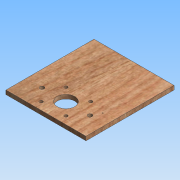
# Autodesk Inventor part: holder_plate
Saved by Autodesk Inventor 2015 (Build 190159000, 159)
## iProperties
Created: 2013-12-24
Part Number: holder_plate
Material: Wood (Birch)
Document SubType Name: Modeling
Designer: aoki
Density: 1 g/cm^3
Appearance: Birch - Natural Polished
Author: aoki
Autodesk Inventor part; units mm, degrees
ref_plane "YZ Plane" through (0, 0, 0) normal (1, 0, 0) x (0, 1, 0)
ref_plane "XZ Plane" through (0, 0, 0) normal (0, 1, 0) x (-1, 0, 0)
ref_plane "XY Plane" through (0, 0, 0) normal (0, 0, 1) x (1, 0, 0)
sketch "Block1" plane through (0, 0, 0) normal (0, 0, 1) x (1, 0, 0)
  line L0 (-30.1, 34.1) -> (-9.9, 34.1)
  line L1 (-9.9, 34.1) -> (-9.9, 25.1)
  line L2 (-9.9, 25.1) -> (9.9, 25.1)
  line L3 (9.9, 25.1) -> (9.9, 34.1)
  line L4 (9.9, 34.1) -> (30.1, 34.1)
  line L5 (30.1, 34.1) -> (30.1, 25.1)
  line L6 (30.1, 25.1) -> (50.1, 25.1)
  line L7 (50.1, 25.1) -> (50.1, 16.5667)
  line L8 (50.1, 16.5667) -> (41.1, 16.5667)
  line L9 (41.1, 16.5667) -> (41.1, 6.7667)
  line L10 (41.1, 6.7667) -> (50.1, 6.7667)
  line L11 (50.1, 6.7667) -> (50.1, -6.7667)
  line L12 (50.1, -6.7667) -> (41.1, -6.7667)
  line L13 (41.1, -6.7667) -> (41.1, -16.5667)
  line L14 (41.1, -16.5667) -> (50.1, -16.5667)
  line L15 (50.1, -16.5667) -> (50.1, -25.1)
  line L16 (50.1, -25.1) -> (30.1, -25.1)
  line L17 (30.1, -25.1) -> (30.1, -34.1)
  line L18 (30.1, -34.1) -> (9.9, -34.1)
  line L19 (9.9, -34.1) -> (9.9, -25.1)
  line L20 (9.9, -25.1) -> (-9.9, -25.1)
  line L21 (-9.9, -25.1) -> (-9.9, -34.1)
  line L22 (-9.9, -34.1) -> (-30.1, -34.1)
  line L23 (-30.1, -34.1) -> (-30.1, -25.1)
  line L24 (-30.1, -25.1) -> (-50.1, -25.1)
  line L25 (-50.1, -25.1) -> (-50.1, -16.5667)
  line L26 (-50.1, -16.5667) -> (-41.1, -16.5667)
  line L27 (-41.1, -16.5667) -> (-41.1, -6.7667)
  line L28 (-41.1, -6.7667) -> (-50.1, -6.7667)
  line L29 (-50.1, -6.7667) -> (-50.1, 6.7667)
  line L30 (-50.1, 6.7667) -> (-41.1, 6.7667)
  line L31 (-41.1, 6.7667) -> (-41.1, 16.5667)
  line L32 (-41.1, 16.5667) -> (-50.1, 16.5667)
  line L33 (-50.1, 16.5667) -> (-50.1, 25.1)
  line L34 (-50.1, 25.1) -> (-30.1, 25.1)
  line L35 (-30.1, 25.1) -> (-30.1, 34.1)
  circle A0 centre (-30, 0) radius 4.6
  circle A1 centre (-15.5, 15.5) radius 2.1
  circle A2 centre (-15.5, -15.5) radius 2.1
  circle A3 centre (0, 0) radius 11.1
  circle A4 centre (15.5, 15.5) radius 2.1
  circle A5 centre (30, 0) radius 4.6
  circle A6 centre (15.5, -15.5) radius 2.1
  point P0 (0, 0)
sketch "Block2" plane through (0, 0, 0) normal (0, 0, 1) x (1, 0, 0)
  line L0 (9.8, 34.2) -> (30.2, 34.2)
  line L1 (30.2, 34.2) -> (30.2, 25.2)
  line L2 (30.2, 25.2) -> (50.2, 25.2)
  line L3 (50.2, 25.2) -> (50.2, 16.4667)
  line L4 (50.2, 16.4667) -> (41.2, 16.4667)
  line L5 (41.2, 16.4667) -> (41.2, 6.8667)
  line L6 (41.2, 6.8667) -> (50.2, 6.8667)
  line L7 (50.2, 6.8667) -> (50.2, -6.8667)
  line L8 (50.2, -6.8667) -> (41.2, -6.8667)
  line L9 (41.2, -6.8667) -> (41.2, -16.4667)
  line L10 (41.2, -16.4667) -> (50.2, -16.4667)
  line L11 (50.2, -16.4667) -> (50.2, -25.2)
  line L12 (50.2, -25.2) -> (30.2, -25.2)
  line L13 (30.2, -25.2) -> (30.2, -34.2)
  line L14 (30.2, -34.2) -> (9.8, -34.2)
  line L15 (9.8, -34.2) -> (9.8, -25.2)
  line L16 (9.8, -25.2) -> (-9.8, -25.2)
  line L17 (-9.8, -25.2) -> (-9.8, -34.2)
  line L18 (-9.8, -34.2) -> (-30.2, -34.2)
  line L19 (-30.2, -34.2) -> (-30.2, -25.2)
  line L20 (-30.2, -25.2) -> (-50.2, -25.2)
  line L21 (-50.2, -25.2) -> (-50.2, -16.4667)
  line L22 (-50.2, -16.4667) -> (-41.2, -16.4667)
  line L23 (-41.2, -16.4667) -> (-41.2, -6.8667)
  line L24 (-41.2, -6.8667) -> (-50.2, -6.8667)
  line L25 (-50.2, -6.8667) -> (-50.2, 6.8667)
  line L26 (-50.2, 6.8667) -> (-41.2, 6.8667)
  line L27 (-41.2, 6.8667) -> (-41.2, 16.4667)
  line L28 (-41.2, 16.4667) -> (-50.2, 16.4667)
  line L29 (-50.2, 16.4667) -> (-50.2, 25.2)
  line L30 (-50.2, 25.2) -> (-30.2, 25.2)
  line L31 (-30.2, 25.2) -> (-30.2, 34.2)
  line L32 (-30.2, 34.2) -> (-9.8, 34.2)
  line L33 (-9.8, 34.2) -> (-9.8, 25.2)
  line L34 (-9.8, 25.2) -> (9.8, 25.2)
  line L35 (9.8, 25.2) -> (9.8, 34.2)
  circle A0 centre (-15.5, 15.5) radius 2.2
  circle A1 centre (15.5, 15.5) radius 2.2
  circle A2 centre (30, 0) radius 4.7
  circle A3 centre (15.5, -15.5) radius 2.2
  circle A4 centre (-15.5, -15.5) radius 2.2
  circle A5 centre (-30, 0) radius 4.7
  circle A6 centre (0, 0) radius 11.2
  point P0 (0, 0)
sketch "Block3" plane through (0, 0, 0) normal (0, 0, 1) x (1, 0, 0)
  line L0 (9.9, 34.1) -> (30.1, 34.1)
  line L1 (30.1, 34.1) -> (30.1, 25.1)
  line L2 (30.1, 25.1) -> (50.1, 25.1)
  line L3 (50.1, 25.1) -> (50.1, 16.5667)
  line L4 (50.1, 16.5667) -> (41.1, 16.5667)
  line L5 (41.1, 16.5667) -> (41.1, 6.7667)
  line L6 (41.1, 6.7667) -> (50.1, 6.7667)
  line L7 (50.1, 6.7667) -> (50.1, -6.7667)
  line L8 (50.1, -6.7667) -> (41.1, -6.7667)
  line L9 (41.1, -6.7667) -> (41.1, -16.5667)
  line L10 (41.1, -16.5667) -> (50.1, -16.5667)
  line L11 (50.1, -16.5667) -> (50.1, -25.1)
  line L12 (50.1, -25.1) -> (30.1, -25.1)
  line L13 (30.1, -25.1) -> (30.1, -34.1)
  line L14 (30.1, -34.1) -> (9.9, -34.1)
  line L15 (9.9, -34.1) -> (9.9, -25.1)
  line L16 (9.9, -25.1) -> (-9.9, -25.1)
  line L17 (-9.9, -25.1) -> (-9.9, -34.1)
  line L18 (-9.9, -34.1) -> (-30.1, -34.1)
  line L19 (-30.1, -34.1) -> (-30.1, -25.1)
  line L20 (-30.1, -25.1) -> (-50.1, -25.1)
  line L21 (-50.1, -25.1) -> (-50.1, -16.5667)
  line L22 (-50.1, -16.5667) -> (-41.1, -16.5667)
  line L23 (-41.1, -16.5667) -> (-41.1, -6.7667)
  line L24 (-41.1, -6.7667) -> (-50.1, -6.7667)
  line L25 (-50.1, -6.7667) -> (-50.1, 6.7667)
  line L26 (-50.1, 6.7667) -> (-41.1, 6.7667)
  line L27 (-41.1, 6.7667) -> (-41.1, 16.5667)
  line L28 (-41.1, 16.5667) -> (-50.1, 16.5667)
  line L29 (-50.1, 16.5667) -> (-50.1, 25.1)
  line L30 (-50.1, 25.1) -> (-30.1, 25.1)
  line L31 (-30.1, 25.1) -> (-30.1, 34.1)
  line L32 (-30.1, 34.1) -> (-9.9, 34.1)
  line L33 (-9.9, 34.1) -> (-9.9, 25.1)
  line L34 (-9.9, 25.1) -> (9.9, 25.1)
  line L35 (9.9, 25.1) -> (9.9, 34.1)
  circle A0 centre (-15.5, 15.5) radius 2.1
  circle A1 centre (15.5, 15.5) radius 2.1
  circle A2 centre (30, 0) radius 4.6
  circle A3 centre (15.5, -15.5) radius 2.1
  circle A4 centre (-15.5, -15.5) radius 2.1
  circle A5 centre (-30, 0) radius 4.6
  circle A6 centre (0, 0) radius 11.1
  point P0 (0, 0)
sketch "Block4" plane through (0, 0, 0) normal (0, 0, 1) x (1, 0, 0)
  line L0 (-30.08, 30.58) -> (-9.92, 30.58)
  line L1 (-9.92, 30.58) -> (-9.92, 25.08)
  line L2 (-9.92, 25.08) -> (9.92, 25.08)
  line L3 (9.92, 25.08) -> (9.92, 30.58)
  line L4 (9.92, 30.58) -> (30.08, 30.58)
  line L5 (30.08, 30.58) -> (30.08, 25.08)
  line L6 (30.08, 25.08) -> (50.08, 25.08)
  line L7 (50.08, 25.08) -> (50.08, 16.5867)
  line L8 (50.08, 16.5867) -> (44.58, 16.5867)
  line L9 (44.58, 16.5867) -> (44.58, 6.7467)
  line L10 (44.58, 6.7467) -> (50.08, 6.7467)
  line L11 (50.08, 6.7467) -> (50.08, -6.7467)
  line L12 (50.08, -6.7467) -> (44.58, -6.7467)
  line L13 (44.58, -6.7467) -> (44.58, -16.5867)
  line L14 (44.58, -16.5867) -> (50.08, -16.5867)
  line L15 (50.08, -16.5867) -> (50.08, -25.08)
  line L16 (50.08, -25.08) -> (30.08, -25.08)
  line L17 (30.08, -25.08) -> (30.08, -30.58)
  line L18 (30.08, -30.58) -> (9.92, -30.58)
  line L19 (9.92, -30.58) -> (9.92, -25.08)
  line L20 (9.92, -25.08) -> (-9.92, -25.08)
  line L21 (-9.92, -25.08) -> (-9.92, -30.58)
  line L22 (-9.92, -30.58) -> (-30.08, -30.58)
  line L23 (-30.08, -30.58) -> (-30.08, -25.08)
  line L24 (-30.08, -25.08) -> (-50.08, -25.08)
  line L25 (-50.08, -25.08) -> (-50.08, -16.5867)
  line L26 (-50.08, -16.5867) -> (-44.58, -16.5867)
  line L27 (-44.58, -16.5867) -> (-44.58, -6.7467)
  line L28 (-44.58, -6.7467) -> (-50.08, -6.7467)
  line L29 (-50.08, -6.7467) -> (-50.08, 6.7467)
  line L30 (-50.08, 6.7467) -> (-44.58, 6.7467)
  line L31 (-44.58, 6.7467) -> (-44.58, 16.5867)
  line L32 (-44.58, 16.5867) -> (-50.08, 16.5867)
  line L33 (-50.08, 16.5867) -> (-50.08, 25.08)
  line L34 (-50.08, 25.08) -> (-30.08, 25.08)
  line L35 (-30.08, 25.08) -> (-30.08, 30.58)
  circle A0 centre (-30, 0) radius 4.88
  circle A1 centre (30, 0) radius 4.88
  circle A2 centre (15.5, 15.5) radius 2.08
  circle A3 centre (0, 0) radius 11.08
  circle A4 centre (-15.5, 15.5) radius 2.08
  circle A5 centre (-15.5, -15.5) radius 2.08
  circle A6 centre (15.5, -15.5) radius 2.08
  point P0 (0, 0)
sketch "Sketch10" plane through (0, 0, 0) normal (0, 0, 1) x (1, 0, 0)
  line L0 (50, -25) -> (-50, -25)
  line L1 (-50, -25) -> (-50, 25)
  line L2 (-50, 25) -> (50, 25)
  line L3 (50, 25) -> (50, -25)
  line L4 (50, -25) -> (-50, 25) construction
  line L5 (-50, -25) -> (50, 25) construction
  point P0 (0, 0)
  dimension "d21" = 100
  dimension "d22" = 50
  constraints: 12 end point, 2 midpoint, 2 parallel, 1 horizontal, 1 perpendicular
  measures "d21" distance of L1.end L2.end
  measures "d22" distance of L0.end L1.end
extrude "Extrusion2" add sketch "Sketch10" against normal blind 5
sketch "Sketch13" plane through (0, 0, 0) normal (0, 0, 1) x (1, 0, 0)
  line L0 (0, -47.8822) -> (0, 48.5933) projected
  line L1 (-201.8331, 0) -> (92.0889, 0) projected
  point P0 (-15.5, 15.5)
  point P1 (15.5, 15.5)
  point P2 (-15.5, -15.5)
  point P3 (15.5, -15.5)
  dimension "d43" = 31
  dimension "d44" = 31
  constraints: 3 symmetric about line
  measures "d43" distance of point (15.5, 15.5) point (-15.5, 15.5)
  measures "d44" distance of point (-15.5, -15.5) point (-15.5, 15.5)
hole "Hole4" at (-15.5, 15.5, 0) at (15.5, 15.5, 0) at (-15.5, -15.5, 0) at (15.5, -15.5, 0) direction (0, 0, -1) diameter 4 end through all
sketch "Sketch16" plane through (0, 0, -5) normal (0, 0, -1) x (-1, 0, 0)
  line L0 (0, -47.8822) -> (0, 48.5933) projected
  point P0 (0, 0)
  point P1 (-30, 0)
  point P2 (30, 0)
  dimension "d52" = 60
  constraints: 1 symmetric about line
  measures "d52" distance of point (30, 0) point (-30, 0)
hole "Hole5" at (30, 0, -5) at (-30, 0, -5) direction (0, 0, 1) diameter 5.2 end through all
sketch "Sketch17" plane through (0, 0, -5) normal (0, 0, -1) x (-1, 0, 0)
  point P0 (0, 0)
  point P1 (0, 0)
  constraints: 1 coincident
hole "Hole8" at (0, 0, -5) direction (0, 0, 1) diameter 22 end through all
sketch "Sketch33" plane through (0, 0, 0) normal (0, 0, 1) x (1, 0, 0)
  line L0 (-50, 25) -> (50, 25) projected
  line L1 (-50, -25) -> (-50, 25) projected
  line L2 (0, -47.8822) -> (0, 48.5933) projected
  line L3 (-201.8331, 0) -> (92.0889, 0) projected
  line L4 (-30, 25) -> (-10, 25)
  line L5 (-10, 25) -> (-10, 30.5)
  line L6 (-10, 30.5) -> (-30, 30.5)
  line L7 (-30, 30.5) -> (-30, 25)
  line L8 (30, 25) -> (10, 25)
  line L9 (10, 25) -> (10, 30.5)
  line L10 (10, 30.5) -> (30, 30.5)
  line L11 (30, 30.5) -> (30, 25)
  line L12 (-30, -25) -> (-10, -25)
  line L13 (-10, -25) -> (-10, -30.5)
  line L14 (-10, -30.5) -> (-30, -30.5)
  line L15 (-30, -30.5) -> (-30, -25)
  line L16 (10, -25) -> (10, -30.5)
  line L17 (30, -25) -> (10, -25)
  line L18 (10, -30.5) -> (30, -30.5)
  line L19 (30, -30.5) -> (30, -25)
  point P0 (-50, 16.6667)
  dimension "d121" = 20
  dimension "d122" = 5.5
  dimension "d123" = 20
  constraints: 32 end point, 12 symmetric about line, 2 parallel, 2 point on line, 1 horizontal, 1 perpendicular
  measures "d121" distance of L5.end L6.end
  measures "d122" distance of L6.end L4.start
  measures "d123" distance between parallel lines of L1 L7
extrude "Extrusion5" [suppressed]
sketch "Sketch34" plane through (0, 0, -5) normal (0, 0, -1) x (-1, 0, 0)
  line L0 (50, 25) -> (-50, 25) projected
  line L1 (-50, 25) -> (-50, -25) projected
  line L2 (-50, 16.6667) -> (-44.5, 16.6667)
  line L3 (-44.5, 16.6667) -> (-44.5, 6.6667)
  line L4 (-44.5, 6.6667) -> (-50, 6.6667)
  line L5 (-50, 6.6667) -> (-50, 16.6667)
  line L6 (201.8331, 0) -> (-92.0889, 0) projected
  line L7 (0, -47.8822) -> (0, 48.5933) projected
  line L8 (-50, -16.6667) -> (-44.5, -16.6667)
  line L9 (-44.5, -16.6667) -> (-44.5, -6.6667)
  line L10 (-44.5, -6.6667) -> (-50, -6.6667)
  line L11 (-50, -6.6667) -> (-50, -16.6667)
  line L12 (50, 16.6667) -> (44.5, 16.6667)
  line L13 (44.5, 16.6667) -> (44.5, 6.6667)
  line L14 (44.5, 6.6667) -> (50, 6.6667)
  line L15 (50, 6.6667) -> (50, 16.6667)
  line L16 (44.5, -16.6667) -> (44.5, -6.6667)
  line L17 (50, -16.6667) -> (44.5, -16.6667)
  line L18 (44.5, -6.6667) -> (50, -6.6667)
  line L19 (50, -6.6667) -> (50, -16.6667)
  point P0 (-30, 25)
  dimension "d131" = 5.5
  dimension "d132" = 10
  dimension "d133" = 8.3333
  constraints: 32 end point, 12 symmetric about line, 2 parallel, 1 horizontal, 1 perpendicular, 1 point on line
  measures "d131" distance of L2.start L2.end
  measures "d132" distance of L2.end L3.end
  measures "d133" distance between parallel lines of L0 L2
extrude "Extrusion6" [suppressed]
sketch "Sketch45" plane through (0, 0, 0) normal (0, 0, 1) x (1, 0, 0)
  circle A0 centre (0, 0) radius 11 projected
  circle A1 centre (30, 0) radius 2.6 projected
  circle A2 centre (-30, 0) radius 2.6 projected
  circle A3 centre (-15.5, -15.5) radius 2 projected
  circle A4 centre (-15.5, 15.5) radius 2 projected
  circle A5 centre (15.5, 15.5) radius 2 projected
  circle A6 centre (15.5, -15.5) radius 2 projected
  line L0 (50, -25) -> (-50, -25) projected
  line L1 (50, 25) -> (50, -25) projected
  line L2 (-50, 25) -> (50, 25) projected
  line L3 (-50, -25) -> (-50, 25) projected
  line L4 (50, 25) -> (-50, 25)
  line L5 (-50, 25) -> (-50, 85)
  line L6 (-50, 85) -> (50, 85)
  line L7 (50, 85) -> (50, 25)
  dimension "d189" = 60
  constraints: 8 end point, 2 parallel, 1 horizontal, 1 perpendicular
  measures "d189" distance of L4.end L5.end
extrude "Extrusion10" add sketch "Sketch45" against normal blind 5 contours L2 L5 L6 L7
equation "\"d121\" = 0.2 * d21"
equation "\"d122\" = Wt"
equation "\"d123\" = 0.2 * d21"
equation "\"d129\" = Wt"
equation "\"d131\" = Wt"
equation "\"d132\" = 0.2 * d22"
equation "\"d133\" = 0.166667 * d22"
equation "\"d134\" = Wt"
equation "\"Wt\" = 5.5"
body "Solid2"
